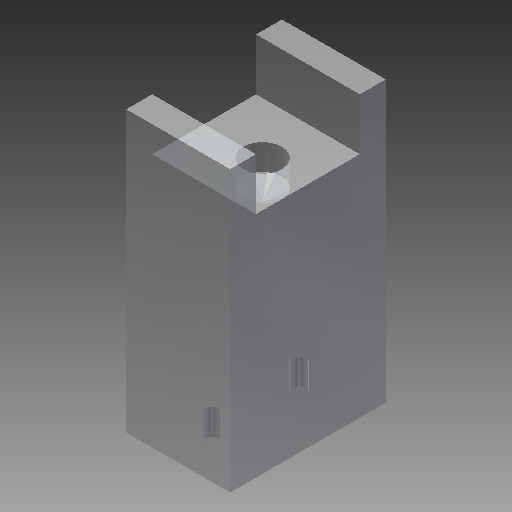
# Autodesk Inventor part: TSV+Support
Saved by Autodesk Inventor 2017 (Build 210142000, 142)
## iProperties
Created: 2017-03-28
Part Number: TSV+Support
Material: Generic
Document SubType Name: Modeling
Designer: hoeflinc
Density: 1 g/cm^3
Appearance: Clear
Quantity: 1
Author: hoeflinc
Autodesk Inventor part; units mm, degrees
ref_plane "YZ Plane" through (0, 0, 0) normal (1, 0, 0) x (0, 1, 0)
ref_plane "XZ Plane" through (0, 0, 0) normal (0, 1, 0) x (-1, 0, 0)
ref_plane "XY Plane" through (0, 0, 0) normal (0, 0, 1) x (1, 0, 0)
sketch "Sketch1" plane through (0, 0, 0) normal (0, 1, 0) x (-1, 0, 0)
  line L0 (0, 0) -> (25.4, 0)
  line L1 (25.4, 0) -> (25.4, -38.1)
  line L2 (25.4, -38.1) -> (0, -38.1)
  line L3 (0, -38.1) -> (0, 0)
  dimension "d0" = 38.1
  dimension "d1" = 25.4
  constraints: 8 end point, 2 parallel, 1 horizontal, 1 perpendicular
  measures "d0" distance of L2.end L0.start
  measures "d1" distance of L0.start L0.end
extrude "Extrusion1" add sketch "Sketch1" along normal blind 68.58
sketch "Sketch2" plane through (0, 68.58, 0) normal (0, 1, 0) x (1, 0, 0)
  line L0 (0, 0) -> (0, 38.1) projected
  line L1 (-25.4, 38.1) -> (-25.4, 0) projected
  line L2 (0, 6.35) -> (-25.4, 6.35)
  line L3 (-25.4, 6.35) -> (-25.4, 31.75)
  line L4 (-25.4, 31.75) -> (0, 31.75)
  line L5 (0, 31.75) -> (0, 6.35)
  line L6 (-25.4, 0) -> (0, 0) projected
  dimension "d4" = 6.35
  dimension "d5" = 25.4
  constraints: 8 end point, 2 parallel, 2 point on line, 1 horizontal, 1 perpendicular
  measures "d4" distance between parallel lines of L6 L2
  measures "d5" distance between parallel lines of L2 L4
extrude "Extrusion2" cut sketch "Sketch2" against normal blind 12.7 contours L2 L1 L4 L0
sketch "Sketch3" plane through (0, 55.88, 0) normal (0, 1, 0) x (1, 0, 0)
  circle A0 centre (-11.1125, 19.05) radius 6.35 projected
  point P0 (0, 0)
  constraints: 1 coincident
hole "Hole1" at (-11.1125, 55.88, -19.05) direction (0, -1, 0) diameter 9.525 depth 6.35 tip angle 118
sketch "Sketch4" plane through (0, 0, 0) normal (0, -1, 0) x (1, 0, 0)
  circle A0 centre (-11.1125, -19.05) radius 4.7625 projected
  line L0 (-25.4, 0) -> (-25.4, -38.1) projected
  line L1 (0, -38.1) -> (0, 0) projected
  line L2 (-25.4, -38.1) -> (0, -38.1) projected
  line L3 (0, 0) -> (-25.4, 0) projected
  point P0 (-12.7, -29.6333)
  point P1 (-12.7, -8.4667)
  dimension "d15" = 25.4
  dimension "d16" = 12.7
  dimension "d17" = 12.7
  dimension "d18" = 8.4667
  dimension "d19" = 8.4667
  measures "d15" distance between parallel lines of L0 L1
  measures "d16" distance from line of L0 point (-12.7, -8.467)
  measures "d17" distance from line of L0 point (-12.7, -29.633)
  measures "d18" distance from line of point (-12.7, -29.633) L2
  measures "d19" distance from line of point (-12.7, -8.467) L3
hole "Hole2" at (-12.7, 0, -29.6333) at (-12.7, 0, -8.4667) direction (0, 1, 0) diameter 3.5052 depth 6.35 tip angle 118
equation "\"d16\" = 0.5 * d15"
equation "\"d17\" = d16"
equation "\"d19\" = d18"
body "Solid1"
